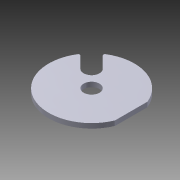
# Autodesk Inventor part: EndCap 108
Saved by Autodesk Inventor 2015 (Build 190159000, 159)
## iProperties
Created: 2011-09-29
Part Number: EndCap 108
Document SubType Name: Modeling
Designer: user
Density: 1 g/cm^3
Material: Generic
Appearance: Cool White
Author: user
Autodesk Inventor part; units mm, degrees
ref_plane "YZ Plane" through (0, 0, 0) normal (1, 0, 0) x (0, 1, 0)
ref_plane "XZ Plane" through (0, 0, 0) normal (0, 1, 0) x (-1, 0, 0)
ref_plane "XY Plane" through (0, 0, 0) normal (0, 0, 1) x (1, 0, 0)
sketch "Sketch1" plane through (0, 0, 0) normal (0, 0, 1) x (1, 0, 0)
  circle A0 centre (0, 0) radius 10
  arc A1 (-28.2843, 14.1421) -> (-14.1421, 28.2843) centre (-21.2132, 21.2132) ccw
  line L0 (-14.1421, 28.2843) -> (-28.706, 42.8482)
  line L1 (-28.2843, 14.1421) -> (-42.8482, 28.706)
  line L2 (50, -20) -> (50, 20)
  arc A2 (-45.9648, 28.3415) -> (49.8462, -20.7692) centre (0, 0) ccw
  arc A3 (49.8462, 20.7692) -> (-28.3415, 45.9648) centre (0, 0) ccw
  arc A4 (-42.8482, 28.706) -> (-45.9648, 28.3415) centre (-44.2624, 27.2918) ccw
  arc A5 (-28.3415, 45.9648) -> (-28.706, 42.8482) centre (-27.2918, 44.2624) ccw
  arc A6 (50, 20) -> (49.8462, 20.7692) centre (48, 20) ccw
  arc A7 (49.8462, -20.7692) -> (50, -20) centre (48, -20) ccw
  line L3 (0, 0) -> (-40.4458, 40.4458) construction
  point P0 (-30.4523, 44.5944)
  point P1 (-44.5944, 30.4523)
  point P2 (50, -20.3961)
  point P3 (50, 20.3961)
  dimension "d1" = 20
  dimension "d4" = 20
  dimension "d12" = 50
  dimension "d13" = 2
  dimension "d14" = 54
  dimension "d15" = 54
  dimension "d16" = 20
  dimension "d19" = 45
  dimension "d21" = 10
  dimension "d22" = 30
  constraints: 19 point on circle, 9 tangent, 8 centre point, 8 end point, 5 point on line, 3 equal radius, 2 coincident, 2 parallel, 1 vertical
  measures "d1" diameter of A0
  measures "d4" diameter of A1
  measures "d12" distance from line of point (0, 0) L2
  measures "d13" radius of A4
  measures "d14" radius of A2
  measures "d15" radius of A3
  measures "d16" distance between parallel lines of L0 L1
  measures "d19" angle of L0 L2
  measures "d21" distance between parallel lines of L0 L3
  measures "d22" distance of A1.centre point (0, 0)
extrude "Extrusion3" add sketch "Sketch1" along normal blind 6
body "Solid3"
